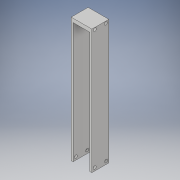
# Autodesk Inventor part: Part11
Saved by Autodesk Inventor 2019 (Build 230136000, 136)
## iProperties
Created: 2018-09-18
Part Number: Part11
Material: Generic
Document SubType Name: Modeling
Designer: drawing
Density: 1 g/cm^3
Appearance: Default
Author: drawing
Autodesk Inventor part; units mm, degrees
ref_plane "YZ Plane" through (0, 0, 0) normal (1, 0, 0) x (0, 1, 0)
ref_plane "XZ Plane" through (0, 0, 0) normal (0, 1, 0) x (-1, 0, 0)
ref_plane "XY Plane" through (0, 0, 0) normal (0, 0, 1) x (1, 0, 0)
sketch "Sketch1" plane through (0, 0, 0) normal (0, 0, 1) x (1, 0, 0)
  line L0 (0, 0) -> (28.575, 0)
  line L1 (28.575, 0) -> (28.575, 203.2)
  line L2 (28.575, 203.2) -> (0, 203.2)
  line L3 (0, 203.2) -> (0, 0)
  line L4 (31.75, 209.55) -> (31.75, 0)
  line L5 (-3.175, 0) -> (-3.175, 209.55)
  line L6 (-3.175, 209.55) -> (31.75, 209.55)
  line L7 (-3.175, 0) -> (31.75, 0)
  dimension "d0" = 28.575
  dimension "d1" = 203.2
  dimension "d2" = 3.175
  dimension "d24" = 6.35
  dimension "d25" = 3.175
  constraints: 16 end point, 3 parallel, 1 horizontal, 1 perpendicular, 1 point on line
  measures "d0" distance of L2.end L1.end
  measures "d1" distance of L1.end L0.end
  measures "d2" distance between parallel lines of L1 L4
  measures "d24" distance between parallel lines of L2 L6
  measures "d25" distance between parallel lines of L3 L5
extrude "Extrusion1" add sketch "Sketch1" along normal blind 28.575 contours L7 L5 L6 L4 L1 L2 L3
sketch "Sketch2" plane through (31.75, 0, 0) normal (1, 0, 0) x (0, 0, -1)
  line L0 (0, 0) -> (-28.575, 0) projected
  line L1 (0, 209.55) -> (0, 0) projected
  point P0 (-23.8125, 5.207)
  point P1 (-4.7625, 5.207)
  dimension "d5" = 5.207
  dimension "d6" = 19.05
  dimension "d7" = 28.575
  dimension "d8" = 4.7625
  constraints: 1 horizontal alignment
  measures "d5" distance from line of point (-4.762, 5.207) L0
  measures "d6" distance of point (-23.812, 5.207) point (-4.762, 5.207)
  measures "d7" distance of L0.start L0.end
  measures "d8" distance from line of L1 point (-4.762, 5.207)
hole "Hole1" at (31.75, 5.207, 23.8125) at (31.75, 5.207, 4.7625) direction (-1, 0, 0) diameter 5.1054 end through all clearance for "Flat Head Machine Screw (82)" size "#10" standard "Ansi Unified Screw Threads"
sketch "Sketch4" plane through (31.75, 0, 0) normal (1, 0, 0) x (0, 0, -1)
  line L0 (-28.575, 0) -> (-28.575, 209.55) projected
  line L1 (0, 209.55) -> (0, 0) projected
  point P0 (-23.495, 206.2387)
  point P1 (-5.08, 206.2387)
  dimension "d26" = 5.08
  dimension "d27" = 5.08
  dimension "d28" = 18.415
  measures "d26" distance from line of L0 point (-23.495, 206.239)
  measures "d27" distance from line of L1 point (-5.08, 206.239)
  measures "d28" distance of point (-23.495, 206.239) point (-5.08, 206.239)
hole "Hole3" at (31.75, 206.2387, 23.495) at (31.75, 206.2387, 5.08) direction (-1, 0, 0) diameter 5.08 depth 10.9728 tip angle 118
equation "\"d8\" = -0.5 * d6 + 0.5 * d7"
equation "\"d27\" = d26"
body "Solid1"
